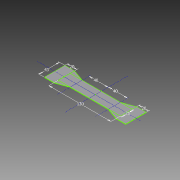
# Autodesk Inventor part: BandMiddle
Saved by Autodesk Inventor 2016 (Build 200138000, 138)
## iProperties
Created: 2015-04-10
Part Number: BandMiddle
Material: Generic
Document SubType Name: Modeling
Designer: Erin
Density: 1 g/cm^3
Appearance: Default
Author: Erin
Autodesk Inventor part; units mm, degrees
ref_plane "YZ Plane" through (0, 0, 0) normal (1, 0, 0) x (0, 1, 0)
ref_plane "XZ Plane" through (0, 0, 0) normal (0, 1, 0) x (-1, 0, 0)
ref_plane "XY Plane" through (0, 0, 0) normal (0, 0, 1) x (1, 0, 0)
sketch "Sketch1" plane through (0, 0, 0) normal (0, 0, 1) x (1, 0, 0)
  line L0 (-65, 12.5) -> (65, 12.5)
  line L1 (65, 12.5) -> (65, -12.5)
  line L2 (65, -12.5) -> (-65, -12.5)
  line L3 (-65, -12.5) -> (-65, 12.5)
  line L4 (-65, 12.5) -> (-65, 21.5)
  line L5 (-65, -12.5) -> (-65, -21.5)
  line L6 (65, 12.5) -> (65, 21.5)
  line L7 (65, -12.5) -> (65, -21.5)
  line L8 (-65, 21.5) -> (-40, 12.5)
  line L9 (-65, -21.5) -> (-40, -12.5)
  line L10 (40, -12.5) -> (65, -21.5)
  line L11 (40, 12.5) -> (65, 21.5)
  line L12 (65, -10.7019) -> (65, -12.5)
  line L13 (-40, 30.8502) -> (-40, -39.2706) construction
  line L14 (40, 30.8502) -> (40, -39.2706) construction
  line L15 (-122.9274, 0) -> (95.3205, 0) construction
  line L16 (0, 69.381) -> (0, -63.5203) construction
  line L17 (-65, 21.5) -> (-85, 21.5)
  line L18 (-85, 21.5) -> (-85, -21.5)
  line L19 (-85, -21.5) -> (-65, -21.5)
  line L20 (-65, -21.5) -> (-65, 21.5)
  line L21 (65, 21.5) -> (85, 21.5)
  line L22 (85, 21.5) -> (85, -21.5)
  line L23 (85, -21.5) -> (65, -21.5)
  line L24 (65, -21.5) -> (65, 21.5)
  line L25 (-65, 21.5) -> (-65, -21.5)
  point P0 (0, 0)
  point P1 (0, 0)
  point P2 (-65, 0)
  point P3 (0, 12.5)
  dimension "d0" = 130
  dimension "d1" = 25
  dimension "d2" = 40
  dimension "d3" = 40
  dimension "d4" = 20
  dimension "d5" = 20
  dimension "d15" = 43
  constraints: 52 end point, 11 point on line, 7 parallel, 6 perpendicular, 5 collinear, 4 horizontal, 2 midpoint, 1 horizontal alignment, 1 vertical, 1 vertical alignment
  measures "d0" distance of L1.end L3.start
  measures "d1" distance of L1.start L1.end
  measures "d2" distance between parallel lines of L13 L16
  measures "d3" distance between parallel lines of L14 L16
  measures "d4" distance of L8.start L17.end
  measures "d5" distance of L6.end L21.end
  measures "d15" distance of L17.end L18.end
extrude "Extrusion1" add sketch "Sketch1" along normal blind 0.2
extrude "Extrusion3" add sketch "Sketch1" along normal blind 0.4 contours L3 L5 L19 L18 L17 L4
mirror "Mirror2" about plane through (0, 0, 0) normal (1, 0, 0) of "Extrusion3"
equation "\"d11\" = material"
equation "\"d16\" = 2 * material"
equation "\"material\" = 0.2"
body "Solid1"
